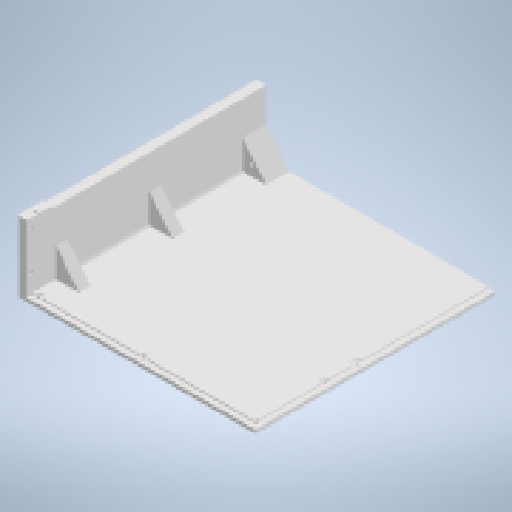
# Autodesk Inventor part: オンゲキボタン_bottom_right1
Saved by Autodesk Inventor 2025.2 (Build 292293000, 293)
## iProperties
Created: 2025-05-16
Part Number: オンゲキボタン_bottom_right1
Material: 一般
Document SubType Name: Modeling
Designer: mahhy
Density: 1 g/cm^3
Appearance: 既定
Author: mahhy
## iProperties of the stored document オンゲキボタン_bottom_right1_3D プリント.ipt
Created: 2025-05-16
Part Number: オンゲキボタン_bottom_right1_3D プリント
Material: 一般
Document SubType Name: Modeling
Designer: mahhy
Density: 1 g/cm^3
Appearance: 既定
Author: mahhy
Autodesk Inventor part; units mm, degrees
ref_plane "YZ Plane" through (0, 0, 0) normal (1, 0, 0) x (0, 1, 0)
ref_plane "XZ Plane" through (0, 0, 0) normal (0, 1, 0) x (-1, 0, 0)
ref_plane "XY Plane" through (0, 0, 0) normal (0, 0, 1) x (1, 0, 0)
sketch "スケッチ1" plane through (0, 0, 0) normal (0, 1, 0) x (-1, 0, 0)
  line L0 (0, 0) -> (204, 0)
  line L1 (204, 0) -> (204, -205)
  line L2 (204, -205) -> (0, -205)
  line L3 (0, -205) -> (0, 0)
  dimension "d0" = 204
  dimension "d1" = 205
  constraints: 8 end point, 2 parallel, 1 horizontal, 1 perpendicular
  measures "d0" distance of L1.end L2.end
  measures "d1" distance of L0.end L1.end
extrude "押し出し1" add sketch "スケッチ1" along normal blind 5
sketch "スケッチ2" plane through (0, 5, 0) normal (0, 1, 0) x (1, 0, 0)
  line L0 (-204, 205) -> (-204, 0) projected
  line L1 (0, 205) -> (-204, 205) projected
  line L2 (-204, 0) -> (-196, 0)
  line L3 (-196, 0) -> (-196, 205)
  line L4 (-196, 205) -> (-204, 205)
  line L5 (-204, 205) -> (-204, 0)
  point P0 (0, 0)
  dimension "d4" = 8
  constraints: 8 end point, 2 parallel, 1 horizontal, 1 perpendicular, 1 point on line
  measures "d4" distance of L4.end L3.end
extrude "押し出し2" add sketch "スケッチ2" along normal blind 56
sketch "スケッチ3" plane through (0, 61, 0) normal (0, 1, 0) x (1, 0, 0)
  circle A0 centre (-198.5, 10) radius 1.5
  line L0 (-204, 0) -> (-196, 0) projected
  line L1 (-204, 205) -> (-204, 0) projected
  point P0 (0, 0)
  dimension "d7" = 3
  dimension "d8" = 10
  dimension "d9" = 5.5
  constraints: 1 centre point
  measures "d7" diameter of A0
  measures "d8" distance from line of L0 A0.centre
  measures "d9" distance from line of L1 A0.centre
extrude "押し出し3" cut sketch "スケッチ3" against normal blind 12
sketch "スケッチ4" plane through (-204, 0, -205) normal (-1, 0, 0) x (0, 0, 1)
  circle A0 centre (201, 20) radius 1.5
  circle A1 centre (201, 53) radius 1.5
  line L0 (0, 0) -> (205, 0) projected
  line L1 (205, 0) -> (205, 61) projected
  dimension "d12" = 3
  dimension "d13" = 3
  dimension "d14" = 20
  dimension "d15" = 33
  dimension "d18" = 4
  constraints: 2 centre point, 1 vertical alignment
  measures "d12" diameter of A0
  measures "d13" diameter of A1
  measures "d14" distance from line of L0 A0.centre
  measures "d15" distance of A0.centre A1.centre
  measures "d18" distance from line of L1 A1.centre
extrude "押し出し4" cut sketch "スケッチ4" against normal through all
sketch "スケッチ5" plane through (-204, 0, -205) normal (-1, 0, 0) x (0, 0, 1)
  circle A0 centre (201, 53) radius 1.5 projected
  circle A1 centre (201, 53) radius 2.8
  circle A2 centre (201, 20) radius 1.5 projected
  circle A3 centre (201, 20) radius 2.8
  point P0 (205, 0)
  dimension "d19" = 5.6
  dimension "d20" = 5.6
  constraints: 2 centre point, 2 coincident
  measures "d19" diameter of A1
  measures "d20" diameter of A3
extrude "押し出し5" cut sketch "スケッチ5" against normal blind 2.5
sketch "スケッチ7" plane through (0, 0, 0) normal (0, -1, 0) x (1, 0, 0)
  circle A0 centre (-5, -5) radius 1.5
  circle A1 centre (-191, -5) radius 1.5
  circle A2 centre (-101, -5) radius 1.5
  circle A3 centre (-5, -64) radius 1.5
  line L0 (-204, 0) -> (0, 0) projected
  line L1 (0, 0) -> (0, -205) projected
  circle A4 centre (-5, -92) radius 1.5
  dimension "d23" = 3
  dimension "d24" = 3
  dimension "d25" = 3
  dimension "d26" = 3
  dimension "d27" = 5
  dimension "d28" = 5
  dimension "d29" = 96
  dimension "d30" = 90
  dimension "d31" = 59
  dimension "d32" = 3
  dimension "d33" = 28
  constraints: 5 centre point, 2 horizontal alignment, 2 vertical alignment
  measures "d23" diameter of A0
  measures "d24" diameter of A1
  measures "d25" diameter of A2
  measures "d26" diameter of A3
  measures "d27" distance from line of L0 A0.centre
  measures "d28" distance from line of L1 A0.centre
  measures "d29" distance of A2.centre A0.centre
  measures "d30" distance of A2.centre A1.centre
  measures "d31" distance of A3.centre A0.centre
  measures "d32" diameter of A4
  measures "d33" distance of A4.centre A3.centre
extrude "押し出し6" cut sketch "スケッチ7" against normal through all
sketch "スケッチ8" plane through (0, 0, 0) normal (0, -1, 0) x (1, 0, 0)
  circle A0 centre (-191, -5) radius 1.5 projected
  circle A1 centre (-191, -5) radius 2.8
  circle A2 centre (-101, -5) radius 1.5 projected
  circle A3 centre (-101, -5) radius 2.8
  circle A4 centre (-5, -5) radius 1.5 projected
  circle A5 centre (-5, -5) radius 2.8
  circle A6 centre (-5, -64) radius 1.5 projected
  circle A7 centre (-5, -64) radius 2.8
  circle A8 centre (-5, -92) radius 1.5 projected
  circle A9 centre (-5, -92) radius 2.8
  point P0 (0, 0)
  dimension "d36" = 5.6
  dimension "d37" = 5.6
  dimension "d38" = 5.6
  dimension "d39" = 5.6
  dimension "d40" = 5.6
  constraints: 5 centre point, 5 coincident
  measures "d36" diameter of A1
  measures "d37" diameter of A3
  measures "d38" diameter of A5
  measures "d39" diameter of A7
  measures "d40" diameter of A9
extrude "押し出し7" cut sketch "スケッチ8" against normal blind 2.5
fillet "フィレット1" radius 1.5 3 edges at (-102, 0, 0) (-204, 0, -102.5) (0, 0, -102.5)
sketch "スケッチ9" plane through (0, 5, 0) normal (0, 1, 0) x (1, 0, 0)
  line L0 (0, 205) -> (-196, 205) projected
  line L1 (0, 205) -> (-5, 205)
  line L2 (-5, 205) -> (-5, 0)
  line L3 (-5, 0) -> (0, 0)
  line L4 (0, 0) -> (0, 205)
  circle A0 centre (-5, 92) radius 2.8 projected
  circle A1 centre (-5, 92) radius 4
  circle A2 centre (-5, 5) radius 1.5 projected
  circle A3 centre (-5, 5) radius 3.1
  circle A4 centre (-5, 64) radius 1.5 projected
  circle A5 centre (-5, 64) radius 3.1
  circle A6 centre (-101, 5) radius 1.5 projected
  circle A7 centre (-101, 5) radius 3.1
  line L5 (-196, 205) -> (-196, 0) projected
  line L6 (0, 0) -> (-196, 0)
  line L7 (-196, 5) -> (0, 5)
  line L8 (0, 5) -> (0, 0)
  line L9 (-196, 0) -> (-186, 0)
  line L10 (-186, 0) -> (-186, 8)
  line L11 (-186, 8) -> (-196, 8)
  line L12 (-196, 8) -> (-196, 0)
  point P0 (-191, 5)
  point P1 (-5, 96)
  point P2 (-5, 88)
  point P3 (-5, 67.1)
  point P4 (-5, 60.9)
  point P5 (-5, 8.1)
  point P6 (-8.1, 5)
  point P7 (-97.9, 5)
  point P8 (-104.1, 5)
  point P9 (-196, 0)
  point P10 (-5, 0)
  point P11 (-5, 5)
  point P12 (-1.9, 5)
  point P13 (-5, 1.9)
  point P14 (-5, 0)
  point P15 (-186, 5)
  point P16 (-196, 8)
  dimension "d44" = 5
  dimension "d45" = 8
  dimension "d46" = 6.2
  dimension "d47" = 6.2
  dimension "d48" = 6.2
  dimension "d50" = 5
  dimension "d83" = 10
  dimension "d84" = 8
  constraints: 22 end point, 5 coincident, 5 parallel, 4 centre point, 3 horizontal, 2 perpendicular, 1 point on line
  measures "d44" distance between parallel lines of L2 L4
  measures "d45" diameter of A1
  measures "d46" diameter of A3
  measures "d47" diameter of A5
  measures "d48" diameter of A7
  measures "d50" distance between parallel lines of L3 L7
  measures "d83" distance of L11.end L10.end
  measures "d84" distance of L10.end L9.end
extrude "押し出し8" cut sketch "スケッチ9" against normal blind 1 contours L4 L7 A3 L2 A5 A1 L0 | L4 L3 L2 A3 L7 | A1 L2 A0 | L2 A0 A1 | L7 A2 L2 A3 | A3 L2 A2 L7 | L11 L10 L7 L5 | A0 L2 | L2 A0 | L6 L10 L7 A7 A3 L2 | L2 A2 L7 A3 | A3 L7 A2 L2 | L7 L2 A2 | A2 L2 L7 | L7 L10 L6 L5 | A5 L2 A4 | L2 A4 A5 | L2 L7 A2 | A2 L7 L2 | A4 L2 | L2 A4 | L7 A6 A7 | A7 L7 A6 | L7 A6 | A6 L7
fillet "フィレット2" radius 2 4 edges at (-203.5607, 0.4393, -0.4393) (-204, 31.25, 0) (-0.4393, 0.4393, -0.4393) (0, 2.75, 0)
sketch "スケッチ10" plane through (0, 5, 0) normal (0, 1, 0) x (1, 0, 0)
  line L0 (-196, 0) -> (-196, 205) projected
  line L1 (-196, 205) -> (-176, 205)
  line L2 (-176, 205) -> (-176, 185)
  line L3 (-176, 185) -> (-196, 185)
  line L4 (-196, 185) -> (-196, 205)
  line L5 (-196, 115) -> (-176, 115)
  line L6 (-176, 115) -> (-176, 105)
  line L7 (-176, 105) -> (-196, 105)
  line L8 (-196, 105) -> (-196, 115)
  line L9 (-196, 25) -> (-176, 25)
  line L10 (-176, 25) -> (-176, 35)
  line L11 (-176, 35) -> (-196, 35)
  line L12 (-196, 35) -> (-196, 25)
  line L13 (0, 205) -> (-196, 205) projected
  point P0 (0, 0)
  point P1 (-5, 205)
  point P2 (-196, 35)
  dimension "d56" = 20
  dimension "d57" = 20
  dimension "d58" = 20
  dimension "d59" = 10
  dimension "d60" = 20
  dimension "d61" = 10
  dimension "d63" = 70
  dimension "d64" = 70
  constraints: 24 end point, 6 parallel, 3 horizontal, 3 perpendicular, 2 point on line
  measures "d56" distance of L2.end L3.end
  measures "d57" distance of L1.end L2.end
  measures "d58" distance of L6.end L7.end
  measures "d59" distance of L5.end L6.end
  measures "d60" distance of L11.end L10.end
  measures "d61" distance of L10.end L9.end
  measures "d63" distance between parallel lines of L5 L3
  measures "d64" distance between parallel lines of L11 L7
extrude "押し出し9" add sketch "スケッチ10" along normal blind 25
sketch "スケッチ11" plane through (-176, 5, -205) normal (0, 0, -1) x (1, 0, 0)
  line L0 (-20, -25) -> (-20, -56) projected
  line L1 (-20, -25) -> (0, 0)
  line L2 (0, 0) -> (0, -25) projected
  line L3 (0, 0) -> (0, -25)
  line L4 (0, -25) -> (-20, -25)
  point P0 (176, 5)
  point P1 (15, 0)
  constraints: 6 end point, 1 collinear, 1 perpendicular, 1 other
extrude "押し出し10" cut sketch "スケッチ11" against normal through all
fillet "フィレット3" radius 2 2 edges at (-196, 5, -70) (-196, 5, -150)
sketch "スケッチ12" plane through (-196, 61, -205) normal (0, 0, -1) x (-1, 0, 0)
  circle A0 centre (-8, -47) radius 1.5
  line L0 (0, -54) -> (0, -31) projected
  line L1 (-191, -56) -> (-20, -56) projected
  point P0 (-196, -61)
  point P1 (-196, -56)
  dimension "d70" = 3
  dimension "d71" = 8
  dimension "d72" = 9
  constraints: 1 centre point
  measures "d70" diameter of A0
  measures "d71" distance from line of A0.centre L0
  measures "d72" distance from line of L1 A0.centre
extrude "押し出し11" cut sketch "スケッチ12" against normal blind 25
sketch "スケッチ13" plane through (0, 61, 0) normal (0, 1, 0) x (1, 0, 0)
  line L0 (-204, 205) -> (-202.5, 205) projected
  line L1 (-196, 0) -> (-196, 205) projected
  line L2 (-204, 205) -> (-196, 205)
  line L3 (-196, 205) -> (-196, 22)
  line L4 (-196, 22) -> (-204, 22)
  line L5 (-204, 22) -> (-204, 205)
  point P0 (0, 0)
  dimension "d80" = 183
  constraints: 8 end point, 2 parallel, 1 horizontal, 1 perpendicular, 1 point on line
  measures "d80" distance of L2.end L3.end
extrude "押し出し12" cut sketch "スケッチ13" against normal blind 2
